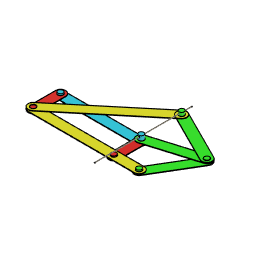
Mechanism v1 (Autodesk Fusion 360 design; units mm, degrees)
Autodesk Fusion 360 part; units mm, degrees
sketch "Sketch1" plane through (0, 0, 0) normal (0, 0, 1) x (1, 0, 0)
  circle A0 centre (-50, 10) radius 5
  circle A1 centre (30, 10) radius 5
  line L0 (-50.0673, 5.0005) -> (31, 5.0005)
  line L1 (31, 14.899) -> (-51, 14.899)
  circle A2 centre (-50, 10) radius 2.5
  circle A3 centre (30, 10) radius 2.5
  dimension "d1" = 10
  dimension "d2" = 10
  dimension "d5" = 5
  dimension "d8" = 5
  constraint coincident A0 L0.start
  constraint horizontal L0
  constraint coincident A1 L1.start
  constraint coincident A0 L1.end
  constraint parallel L0 L1
  constraint concentric A0 A2
  constraint concentric A1 A3
  measures "d1" diameter of A0
  measures "d2" diameter of A1
  measures "d5" diameter of A2
  measures "d8" diameter of A3
extrude "Extrude3" add sketch "Sketch1" along normal blind 3 contours A3 makes body 1
extrude "Extrude1" add sketch "Sketch1" along normal blind 0.5 separate body contours A0 A1 L0 L1 | A0 L1 | A1 L1 | A2 | A3 picked at (-50.0623, 14.097) picked at (30.0623, 14.097) makes body 2
extrude "Extrude2" add sketch "Sketch1" along normal blind 3 contours A2 bodies 2
combine "Combine1" operation add target body 1 tool bodies 2
sketch "Sketch2" plane through (0, 0, 0) normal (0, 0, 1) x (1, 0, 0)
  circle A0 centre (-50, 10) radius 5
  circle A1 centre (-50, -17) radius 5
  line L0 (-45, -17) -> (-45, 11)
  line L1 (-54.899, 11) -> (-54.899, -16)
  circle A2 centre (-50, -17) radius 2.5
  circle A3 centre (-50, 10) radius 2.65
  dimension "d11" = 5
  dimension "d12" = 5.3
  constraint coincident A1 L0.start
  constraint tangent A1 L0
  constraint vertical L0
  constraint coincident A0 L1.start
  constraint coincident A1 L1.end
  constraint parallel L0 L1
  constraint concentric A1 A2
  constraint concentric A0 A3
  measures "d11" diameter of A2
  measures "d12" diameter of A3
extrude "Extrude4" add sketch "Sketch2" along normal blind 0.5 separate body contours A0 L1 | A0 A1 L0 L1 | A1 picked at (-54.1493, 10) makes body 3
extrude "Extrude5" add sketch "Sketch2" along normal blind 3 contours A2 bodies 3
copy_body "Body->Comp1" bodies 3 removing the originals makes body 4 in component "red"
copy_body "Body->Comp2" bodies 1 removing the originals makes body 5 in component "blue base"
sketch "Sketch3" plane through (0, 0, 0) normal (0, 0, 1) x (1, 0, 0)
  circle A0 centre (-50, -17) radius 5
  circle A1 centre (30, -17) radius 5
  circle A2 centre (55, -17) radius 5
  line L0 (-50, -12) -> (55, -12)
  line L1 (55, -22) -> (-50, -22)
  circle A3 centre (-50, -17) radius 2.65
  circle A4 centre (30, -17) radius 2.65
  circle A5 centre (55, -17) radius 2.65
  dimension "d17" = 10
  dimension "d18" = 10
  dimension "d19" = 5.3
  dimension "d20" = 5.3
  dimension "d21" = 5.3
  constraint coincident A0 L0.start
  constraint coincident A2 L0.end
  constraint tangent A2 L0
  constraint coincident A2 L1.start
  constraint coincident A0 L1.end
  constraint tangent A0 L1
  constraint concentric A0 A3
  constraint concentric A1 A4
  constraint concentric A2 A5
  measures "d17" diameter of A1
  measures "d18" diameter of A2
  measures "d19" diameter of A3
  measures "d20" diameter of A4
  measures "d21" diameter of A5
extrude "Extrude1'" add sketch "Sketch3" along normal blind 0.5 separate body makes body 6 in component "down yellow"
sketch "Sketch4" plane through (0, 0, 0) normal (0, 0, 1) x (1, 0, 0)
  circle A0 centre (54.992, -16.9822) radius 4.958
  circle A1 centre (80, 25) radius 5
  line L0 (84.3763, 22.5818) -> (59.2495, -19.5229)
  line L1 (51.2473, -13.7327) -> (76.4824, 28.5534)
  circle A2 centre (54.992, -16.9822) radius 2.5
  circle A3 centre (80, 25) radius 2.5
  dimension "d24" = 10
  dimension "d25" = 5
  dimension "d26" = 5
  constraint coincident A1 L0.start
  constraint coincident A0 L0.end
  constraint tangent A0 L0
  constraint coincident A0 L1.start
  constraint coincident A1 L1.end
  constraint parallel L0 L1
  constraint concentric A0 A2
  constraint concentric A1 A3
  measures "d24" diameter of A1
  measures "d25" diameter of A2
  measures "d26" diameter of A3
extrude "Extrude6" add sketch "Sketch4" along normal blind 0.5 separate body contours A0 | A1 L1 | A0 A1 L0 L1 picked at (76.5398, 27.1235) makes body 7
extrude "Extrude7" add sketch "Sketch4" along normal blind 3 contours A2 | A3 bodies 7
copy_body "Body->Comp3" bodies 7 removing the originals makes body 8 in component "right green"
sketch "Sketch5" plane through (0, 0, 0) normal (0, 0, 1) x (1, 0, 0)
  circle A0 centre (30, 10) radius 5
  circle A1 centre (80, 25) radius 5
  line L0 (28.0625, 14.6093) -> (78.5607, 29.7884)
  line L1 (82.1683, 20.4946) -> (31.4423, 5.2125)
  circle A2 centre (30, 10) radius 2.65
  circle A3 centre (80, 25) radius 2.65
  dimension "d31" = 10
  dimension "d32" = 10
  dimension "d33" = 5.3
  dimension "d34" = 5.3
  constraint coincident A0 L0.start
  constraint coincident A1 L0.end
  constraint tangent A1 L0
  constraint coincident A1 L1.start
  constraint coincident A0 L1.end
  constraint tangent A0 L1
  constraint concentric A0 A2
  constraint concentric A1 A3
  measures "d31" diameter of A0
  measures "d32" diameter of A1
  measures "d33" diameter of A2
  measures "d34" diameter of A3
extrude "Extrude1''" add sketch "Sketch5" along normal blind 0.5 separate body contours A0 L0 | A0 A1 L0 L1 | A1 L1 picked at (28.8493, 14.0355) picked at (81.1464, 20.9859) makes body 9 in component "middle green"
sketch "Sketch6" plane through (0, 0, 0) normal (0, 0, 1) x (1, 0, 0)
  circle A0 centre (80, 25) radius 5
  circle A1 centre (30, 50) radius 5
  line L0 (82.9436, 29.0417) -> (32.056, 54.5577)
  line L1 (77.533, 20.651) -> (27.0449, 45.9667)
  circle A2 centre (80, 25) radius 2.65
  circle A3 centre (30, 50) radius 2.5
  dimension "d37" = 10
  dimension "d38" = 10
  dimension "d39" = 5.3
  dimension "d40" = 5
  constraint coincident A0 L0.start
  constraint coincident A1 L0.end
  constraint coincident A0 L1.start
  constraint coincident A1 L1.end
  constraint parallel L0 L1
  constraint concentric A0 A2
  constraint concentric A1 A3
  measures "d37" diameter of A0
  measures "d38" diameter of A1
  measures "d39" diameter of A2
  measures "d40" diameter of A3
extrude "Extrude8" add sketch "Sketch6" along normal blind 0.5 separate body contours A0 L0 | A0 A1 L0 L1 | A1 L0 L1 picked at (81.9155, 28.7044) makes body 10
extrude "Extrude9" add sketch "Sketch6" along normal blind 3 contours A3 bodies 10
copy_body "Body->Comp4" bodies 10 removing the originals makes body 11 in component "last green"
sketch "Sketch7" plane through (0, 0, 0) normal (0, 0, 1) x (1, 0, 0)
  circle A0 centre (30.1681, 49.7404) radius 5
  circle A1 centre (-49.9867, -16.9755) radius 5
  line L0 (-53.8778, -13.8356) -> (26.9659, 53.5804)
  circle A2 centre (-49.9867, -16.9755) radius 2.65
  line L1 (-46.5205, -20.5791) -> (33.3663, 45.897)
  circle A3 centre (30.1681, 49.7404) radius 2.65
  dimension "d45" = 10
  dimension "d46" = 10
  dimension "d47" = 5.3
  dimension "d48" = 5.3
  constraint coincident A1 L0.start
  constraint coincident A0 L0.end
  constraint tangent A0 L0
  constraint concentric A1 A2
  constraint coincident A1 L1.start
  constraint coincident A0 L1.end
  constraint tangent A0 L1
  constraint concentric A0 A3
  measures "d45" diameter of A0
  measures "d46" diameter of A1
  measures "d47" diameter of A2
  measures "d48" diameter of A3
extrude "Extrude1'''" add sketch "Sketch7" along normal blind 0.5 separate body contours A0 | A0 A1 L0 L1 | A1 L0 picked at (-52.6311, -13.7743) makes body 12 in component "up yellow"
move_face "OffsetFaces1" offset -0.5 1 faces at (-50.7053, -17.2456, 3) on bodies 4 in component "red"
move_face "OffsetFaces1'" offset 4 1 faces at (30.3177, 10.4694, 3) on bodies 5 in component "blue base"
move_face "OffsetFaces1''" offset 1 1 faces at (30.6608, 50.348, 3) on bodies 11 in component "last green"
sketch "Sketch8" plane through (0, 0, 0) normal (0, 1, 0) x (1, 0, 0)
  circle A0 centre (30, -5.5) radius 1
  dimension "d54" = 2
  measures "d54" diameter of A0
extrude "Extrude10" add sketch "Sketch8" against normal blind 31 separate body makes body 13
move_face "OffsetFaces1'''" offset 50 1 faces at (29.9258, 0, 5.175) on bodies 13
copy_body "Body->Comp1'" bodies 5 removing the originals makes body 14 in component "Base body (1)"
copy_body "Body->Comp5" bodies 13 removing the originals makes body 15 in component "Axis"
move_face "OffsetFaces1''''" offset -0.5 1 faces at (30.1736, 23, 6.4848) on bodies 15 in component "Axis"
move_face "OffsetFaces2" offset 15 1 faces at (30.0609, -31, 5.3449) on bodies 15 in component "Axis"
sketch "Sketch9" plane through (0, 0, 0) normal (0, 1, 0) x (1, 0, 0)
  circle A0 centre (30, -5.5) radius 0.65
  dimension "d60" = 1.3
  measures "d60" diameter of A0
extrude "Extrude1''''" cut sketch "Sketch9" along normal blind 14 sketch seen with x (1, 0, 0) y (0, 1, 0) z (0, 0, 1) at (0.1376, -0.2752, 0) bodies 14 in component "Base body (1)"
component "red" placed x (1, 0, 0) y (0, 1, 0) z (0, 0, 1) at (-0.1643, 0.3077, 1.1061)
component "blue base" placed x (1, 0, 0) y (0, 1, 0) z (0, 0, 1) at (-0.1376, 0.2752, 0)
component "red" placed x (1, 0, 0) y (0, 1, 0) z (0, 0, 1) at (79.9321, -0.011, 0.9207)
component "down yellow" placed x (1, 0, 0) y (0, 1, 0) z (0, 0, 1) at (0, 0, 2.1033)
component "right green" placed x (1, 0, 0) y (0, 1, 0) z (0, 0, 1) at (-0.0107, -0.0077, 0.8439)
component "middle green" placed x (1, 0, 0) y (0, 1, 0) z (0, 0, 1) at (-0.0494, 0.2866, 2.2754)
component "last green" placed x (1, 0, 0) y (0, 1, 0) z (0, 0, 1) at (0.0028, 0.0174, 3.1793)
component "up yellow" placed x (1, 0, 0) y (0, 1, 0) z (0, 0, 1) at (-0.1843, 0.2924, 3.398)
component "Axis" placed x (1, 0, 0) y (0, 1, 0) z (0, 0, 1) at (0, 10.0328, 0)
component "Base body (1)" placed x (1, 0, 0) y (0, 1, 0) z (0, 0, 1) at (0, 0, 0) in component "blue base"
named bodies: "Base body", "Left red"
